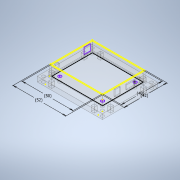
# Autodesk Inventor part: TNC Case
Saved by Autodesk Inventor 2020.1 (Build 241239000, 239)
## iProperties
Created: 2019-09-18
Part Number: TNC Case
Material: PET Plastic
Document SubType Name: Modeling
Designer: Logan
Density: 1.541 g/cm^3
Appearance: Polycarbonate - Clear
Author: Logan
Autodesk Inventor part; units mm, degrees
ref_plane "YZ Plane" through (0, 0, 0) normal (1, 0, 0) x (0, 1, 0)
ref_plane "XZ Plane" through (0, 0, 0) normal (0, 1, 0) x (-1, 0, 0)
ref_plane "XY Plane" through (0, 0, 0) normal (0, 0, 1) x (1, 0, 0)
sketch "Sketch1" plane through (0, 0, 0) normal (0, 1, 0) x (-1, 0, 0)
  line L0 (0, 0) -> (60, 0)
  line L1 (60, 0) -> (60, -50)
  line L2 (60, -50) -> (0, -50)
  line L3 (0, -50) -> (0, 0)
  line L4 (60, 0) -> (0, 0)
  line L5 (0, 0) -> (0, -5)
  line L6 (0, -5) -> (60, -5)
  line L7 (60, -5) -> (60, 0)
  line L8 (60, 0) -> (55, 0)
  line L9 (55, 0) -> (55, -50)
  line L10 (55, -50) -> (60, -50)
  line L11 (60, -50) -> (60, 0)
  line L12 (60, -50) -> (0, -50)
  line L13 (0, -50) -> (0, -45)
  line L14 (0, -45) -> (60, -45)
  line L15 (60, -45) -> (60, -50)
  line L16 (0, -50) -> (5, -50)
  line L17 (5, -50) -> (5, 0)
  line L18 (5, 0) -> (0, 0)
  line L19 (0, 0) -> (0, -50)
  line L20 (5, -5) -> (55, -5)
  line L21 (55, -5) -> (55, -45)
  line L22 (55, -45) -> (5, -45)
  line L23 (5, -45) -> (5, -5)
  dimension "d0" = 60
  dimension "d1" = 50
  dimension "d2" = 5
  dimension "d3" = 5
  dimension "d4" = 5
  dimension "d5" = 5
  dimension "d6" = 40
  dimension "d7" = 50
  constraints: 48 end point, 12 parallel, 8 point on line, 6 horizontal, 6 perpendicular
  measures "d0" distance of L1.end L2.end
  measures "d1" distance of L0.end L1.end
  measures "d2" distance of L5.end L4.end
  measures "d3" distance of L10.end L9.end
  measures "d4" distance of L12.end L13.end
  measures "d5" distance of L18.end L17.end
  measures "d6" distance between parallel lines of L22 L20
  measures "d7" distance between parallel lines of L23 L21
extrude "Extrusion1" add sketch "Sketch1" along normal blind 5
sketch "Sketch2" plane through (0, 5, 0) normal (0, 1, 0) x (1, 0, 0)
  line L0 (-60, 50) -> (-60, 0) projected
  line L1 (0, 50) -> (-60, 50) projected
  line L2 (-60, 0) -> (0, 0)
  line L3 (0, 0) -> (0, 50)
  line L4 (0, 50) -> (-60, 50)
  line L5 (-60, 50) -> (-60, 0)
  line L6 (0, 0) -> (0, 50) projected
  line L7 (-60, 0) -> (0, 0)
  line L8 (0, 0) -> (0, 5)
  line L9 (0, 5) -> (-60, 5)
  line L10 (-60, 5) -> (-60, 0)
  line L11 (0, 50) -> (-60, 50)
  line L12 (-60, 50) -> (-60, 45)
  line L13 (-60, 45) -> (0, 45)
  line L14 (0, 45) -> (0, 50)
  line L15 (-60, 0) -> (0, 0) projected
  line L16 (-60, 50) -> (-55, 50)
  line L17 (-55, 50) -> (-55, 0)
  line L18 (-55, 0) -> (-60, 0)
  line L19 (-60, 0) -> (-60, 50)
  line L20 (0, 0) -> (-5, 0)
  line L21 (-5, 0) -> (-5, 50)
  line L22 (-5, 50) -> (0, 50)
  line L23 (0, 50) -> (0, 0)
  line L24 (-55, 5) -> (-56.5, 5)
  line L25 (-56.5, 5) -> (-56.5, 3.5)
  line L26 (-56.5, 3.5) -> (-55, 3.5)
  line L27 (-55, 3.5) -> (-55, 5)
  line L28 (-60, 0) -> (-62, 0)
  line L29 (-62, 0) -> (-62, 50)
  line L30 (-62, 50) -> (-60, 50)
  line L31 (-60, 50) -> (-60, 0)
  line L32 (-62, 0) -> (0, 0)
  line L33 (0, 0) -> (0, -2)
  line L34 (0, -2) -> (-62, -2)
  line L35 (-62, -2) -> (-62, 0)
  line L36 (-62, 50) -> (2, 50)
  line L37 (2, 50) -> (2, 52)
  line L38 (2, 52) -> (-62, 52)
  line L39 (-62, 52) -> (-62, 50)
  line L40 (2, 50) -> (0, 50)
  line L41 (0, 50) -> (0, -2)
  line L42 (0, -2) -> (2, -2)
  line L43 (2, -2) -> (2, 50)
  dimension "d10" = 5
  dimension "d11" = 5
  dimension "d12" = 5
  dimension "d13" = 5
  dimension "d14" = 1.5
  dimension "d15" = 1.5
  dimension "d16" = 2
  dimension "d17" = 2
  dimension "d18" = 64
  dimension "d19" = 2
  constraints: 80 end point, 20 parallel, 10 horizontal, 10 perpendicular, 8 point on line
  measures "d10" distance of L8.end L7.end
  measures "d11" distance of L12.end L11.end
  measures "d12" distance of L17.end L18.end
  measures "d13" distance of L21.end L22.end
  measures "d14" distance of L26.end L25.end
  measures "d15" distance of L25.end L24.end
  measures "d16" distance of L29.end L30.end
  measures "d17" distance of L32.end L33.end
  measures "d18" distance of L38.end L37.end
  measures "d19" distance of L37.end L36.end
extrude "Extrusion2" add sketch "Sketch2" against normal blind 5 contours L30 L39 L38 L37 L36 L1 | L0 L28 L29 L30 | L28 L2 L33 L34 L35 | L36 L43 L42 L33 L3
sketch "Sketch3" plane through (0, 5, 0) normal (0, 1, 0) x (1, 0, 0)
  line L0 (2, -2) -> (-62, -2) projected
  line L1 (2, 52) -> (2, -2) projected
  line L2 (-62, -2) -> (2, -2)
  line L3 (2, -2) -> (2, 52)
  line L4 (2, 52) -> (-62, 52)
  line L5 (-62, 52) -> (-62, -2)
  line L6 (-62, -2) -> (2, -2)
  line L7 (2, -2) -> (2, 4)
  line L8 (2, 4) -> (-62, 4)
  line L9 (-62, 4) -> (-62, -2)
  line L10 (2, 52) -> (-62, 52)
  line L11 (-62, 52) -> (-62, 46)
  line L12 (-62, 46) -> (2, 46)
  line L13 (2, 46) -> (2, 52)
  line L14 (-62, -2) -> (-62, 52) projected
  line L15 (-62, 52) -> (-56, 52)
  line L16 (-56, 52) -> (-56, -2)
  line L17 (-56, -2) -> (-62, -2)
  line L18 (-62, -2) -> (-62, 52)
  line L19 (-62, 52) -> (2, 52) projected
  line L20 (2, -2) -> (-4, -2)
  line L21 (-4, -2) -> (-4, 52)
  line L22 (-4, 52) -> (2, 52)
  line L23 (2, 52) -> (2, -2)
  line L24 (-4, 46) -> (-54, 46)
  line L25 (-54, 46) -> (-54, 6)
  line L26 (-54, 6) -> (-4, 6)
  line L27 (-4, 6) -> (-4, 46)
  line L28 (-56, 4) -> (-6, 4)
  line L29 (-6, 4) -> (-6, 44)
  line L30 (-6, 44) -> (-56, 44)
  line L31 (-56, 44) -> (-56, 4)
  line L32 (-56, 4) -> (-5, 4)
  line L33 (-5, 4) -> (-5, 45)
  line L34 (-5, 45) -> (-56, 45)
  line L35 (-56, 45) -> (-56, 4)
  line L36 (-4, 46) -> (-55, 46)
  line L37 (-55, 46) -> (-55, 5)
  line L38 (-55, 5) -> (-4, 5)
  line L39 (-4, 5) -> (-4, 46)
  line L40 (-4, 5) -> (-56, 5)
  line L41 (-56, 5) -> (-56, 4)
  line L42 (-56, 4) -> (-4, 4)
  line L43 (-4, 4) -> (-4, 5)
  line L44 (-56, 4) -> (-55, 4)
  line L45 (-55, 4) -> (-55, 46)
  line L46 (-55, 46) -> (-56, 46)
  line L47 (-56, 46) -> (-56, 4)
  line L48 (-56, 45) -> (-4, 45)
  line L49 (-4, 45) -> (-4, 46)
  line L50 (-4, 46) -> (-56, 46)
  line L51 (-56, 46) -> (-56, 45)
  line L52 (-4, 46) -> (-5, 46)
  line L53 (-5, 46) -> (-5, 4)
  line L54 (-5, 4) -> (-4, 4)
  line L55 (-4, 4) -> (-4, 46)
  point P0 (0, 0)
  point P1 (-4, 4)
  point P2 (-55, 45)
  point P3 (-5, 5)
  point P4 (-55, 5)
  dimension "d22" = 6
  dimension "d23" = 6
  dimension "d24" = 6
  dimension "d25" = 6
  dimension "d26" = 50
  dimension "d27" = 40
  dimension "d28" = 50
  dimension "d29" = 40
  dimension "d30" = 51
  dimension "d31" = 41
  dimension "d32" = 51
  dimension "d33" = 41
  dimension "d34" = 40
  dimension "d35" = 50
  constraints: 104 end point, 26 parallel, 13 horizontal, 13 perpendicular, 8 point on line
  measures "d22" distance of L7.end L6.end
  measures "d23" distance of L11.end L10.end
  measures "d24" distance of L16.end L17.end
  measures "d25" distance of L21.end L22.end
  measures "d26" distance of L26.end L25.end
  measures "d27" distance of L25.end L24.end
  measures "d28" distance of L30.end L29.end
  measures "d29" distance of L29.end L28.end
  measures "d30" distance of L34.end L33.end
  measures "d31" distance of L33.end L32.end
  measures "d32" distance of L38.end L37.end
  measures "d33" distance of L37.end L36.end
  measures "d34" distance between parallel lines of L34 L38
  measures "d35" distance between parallel lines of L33 L37
extrude "Extrusion3" add sketch "Sketch3" along normal blind 10 contours L8 L33 L38 L21 | L16 L40 L45 L8 | L8 L29 L38 L33 | L38 L33 L26 L21 | L21 L48 L53 L12 | L45 L38 L29 L8 | L16 L30 L37 L40 | L26 L33 L48 L21 | L53 L34 L25 L12 | L16 L34 L37 L30 | L25 L34 L37 L12 | L12 L37 L34 L16
sketch "Sketch5" plane through (0, 5, 0) normal (0, 1, 0) x (1, 0, 0)
  line L0 (-55, 5) -> (-55, 45) projected
  line L1 (-55, 45) -> (-5, 45) projected
  line L2 (-55, 5) -> (-5, 5)
  line L3 (-5, 5) -> (-5, 45)
  line L4 (-5, 45) -> (-55, 45)
  line L5 (-55, 45) -> (-55, 5)
  line L6 (-55, 5) -> (-51, 5)
  line L7 (-55, 9) -> (-55, 5)
  circle A0 centre (-51, 9) radius 1.5
  line L8 (-5, 45) -> (-5, 5) projected
  line L9 (-5, 5) -> (-9, 5)
  line L10 (-5, 9) -> (-5, 5)
  line L11 (-5, 45) -> (-9, 45)
  line L12 (-5, 41) -> (-5, 45)
  line L13 (-55, 45) -> (-51, 45)
  line L14 (-55, 41) -> (-55, 45)
  circle A1 centre (-9, 41) radius 1.5
  circle A2 centre (-9, 9) radius 1.5
  point P0 (0, 0)
  constraints: 24 end point, 5 horizontal, 3 centre point, 2 parallel, 1 perpendicular
extrude "Extrusion4" cut sketch "Sketch5" against normal blind 10 contours A0 | A1 | A2
sketch "Sketch6" plane through (-4, 5, -4) normal (1, 0, 0) x (0, 0, -1)
  line L0 (0, 10) -> (1, 10)
  line L1 (1, 10) -> (1, 0)
  line L2 (1, 0) -> (0, 0)
  line L3 (0, 0) -> (0, 10)
  line L4 (41, 10) -> (42, 10)
  line L5 (42, 10) -> (42, 0)
  line L6 (42, 0) -> (41, 0)
  line L7 (41, 0) -> (41, 10)
  line L8 (1, 0) -> (6, 0)
  line L9 (6, 0) -> (6, 2)
  line L10 (1, 2) -> (1, 0)
  line L11 (6, 2) -> (24, 2)
  line L12 (24, 2) -> (24, 0)
  line L13 (24, 0) -> (6, 0)
  line L14 (6, 0) -> (6, 2)
  line L15 (1, 0) -> (41, 0) projected
  line L16 (6, 2) -> (11.05, 2)
  line L17 (11.05, 0) -> (6, 0)
  line L18 (6, 0) -> (6, 2)
  line L19 (24, 0) -> (18.95, 0)
  line L20 (18.95, 2) -> (24, 2)
  line L21 (24, 2) -> (24, 0)
  line L22 (6, 2) -> (15, 2)
  line L23 (15, 2) -> (15, 0)
  line L24 (15, 0) -> (6, 0)
  line L25 (6, 0) -> (6, 2)
  line L26 (24, 0) -> (15, 0)
  line L27 (15, 0) -> (15, 2)
  line L28 (15, 2) -> (24, 2)
  line L29 (24, 2) -> (24, 0)
  line L30 (15, 2) -> (12.525, 2)
  line L31 (12.525, 2) -> (12.525, 0)
  line L32 (12.525, 0) -> (15, 0)
  line L33 (15, 0) -> (15, 2)
  line L34 (15, 2) -> (17.475, 2)
  line L35 (17.475, 2) -> (17.475, 0)
  line L36 (17.475, 0) -> (15, 0)
  line L37 (15, 0) -> (15, 2)
  line L38 (24, 0) -> (24.05, 0)
  line L39 (24.05, 0) -> (24.05, 2)
  line L40 (24, 2) -> (24, 0)
  line L41 (24.05, 2) -> (31.55, 2)
  line L42 (31.55, 2) -> (31.55, 0)
  line L43 (31.55, 0) -> (24.05, 0)
  line L44 (24.05, 0) -> (24.05, 2)
  line L45 (32.05, 2) -> (32.05, 0)
  line L46 (32.05, 0) -> (31.55, 0)
  line L47 (31.55, 0) -> (31.55, 2)
  line L48 (32.05, 0) -> (37.05, 0)
  line L49 (37.05, 0) -> (37.05, 2)
  line L50 (37.05, 2) -> (32.05, 2)
  line L51 (32.05, 2) -> (32.05, 0)
  line L52 (1, 0) -> (1, 10) projected
  line L53 (41, 0) -> (1, 0)
  line L54 (1, 0) -> (1, 1.6)
  line L55 (1, 1.6) -> (41, 1.6)
  line L56 (41, 1.6) -> (41, 0)
  line L57 (37.05, 2) -> (32.05, 2)
  line L58 (32.05, 2) -> (32.05, 1.6)
  line L59 (32.05, 1.6) -> (37.05, 1.6)
  line L60 (37.05, 1.6) -> (37.05, 2)
  line L61 (37.05, 2) -> (32.05, 2)
  line L62 (32.05, 2) -> (32.05, 1.6)
  line L63 (32.05, 1.6) -> (37.05, 1.6)
  line L64 (37.05, 1.6) -> (37.05, 2)
  line L65 (37.05, 1.6) -> (32.05, 1.6)
  line L66 (32.05, 1.6) -> (32.05, 6.6)
  line L67 (32.05, 6.6) -> (37.05, 6.6)
  line L68 (37.05, 6.6) -> (37.05, 1.6)
  line L69 (17.475, 2) -> (12.525, 2)
  line L70 (12.525, 2) -> (12.525, 1.6)
  line L71 (12.525, 1.6) -> (17.475, 1.6)
  line L72 (17.475, 1.6) -> (17.475, 2)
  line L73 (15, 1.6) -> (17.57, 1.6)
  line L74 (17.57, 1.6) -> (17.57, 2)
  line L75 (17.57, 2) -> (15, 2)
  line L76 (15, 2) -> (15, 1.6)
  line L77 (15, 1.6) -> (12.43, 1.6)
  line L78 (12.43, 1.6) -> (12.43, 2)
  line L79 (12.43, 2) -> (15, 2)
  line L80 (15, 2) -> (15, 1.6)
  line L81 (17.57, 1.6) -> (12.43, 1.6)
  line L82 (12.43, 1.6) -> (12.43, 8.15)
  line L83 (12.43, 8.15) -> (17.57, 8.15)
  line L84 (17.57, 8.15) -> (17.57, 1.6)
  line L85 (31.55, 1.6) -> (24.05, 1.6)
  line L86 (24.05, 1.6) -> (24.05, 6.6)
  line L87 (24.05, 6.6) -> (31.55, 6.6)
  line L88 (31.55, 6.6) -> (31.55, 1.6)
  point P0 (-4, -5)
  point P1 (32.05, 2)
  point P2 (37.05, 2)
  point P3 (24.05, 2)
  point P4 (31.55, 2)
  point P5 (12.43, 2)
  point P6 (17.57, 2)
  dimension "d48" = 5.05
  dimension "d53" = 7.5
  dimension "d54" = 0.5
  dimension "d55" = 5
  dimension "d58" = 1.6
  dimension "d59" = 5
  dimension "d60" = 5
  dimension "d61" = 2.57
  dimension "d62" = 2.57
  dimension "d63" = 6.55
  dimension "d64" = 7.5
  constraints: 174 end point, 41 parallel, 22 horizontal, 20 perpendicular, 12 point on line, 1 midpoint, 5 other
  measures "d48" distance of L20.start L20.end
  measures "d53" distance of L42.end L43.end
  measures "d54" distance of L45.end L46.end
  measures "d55" distance of L50.end L49.end
  measures "d58" distance of L53.end L54.end
  measures "d59" distance of L66.end L67.end
  measures "d60" distance of L65.end L66.end
  measures "d61" distance of L75.end L74.end
  measures "d62" distance of L78.end L79.end
  measures "d63" distance of L81.end L82.end
  measures "d64" distance of L86.end L87.end
sketch "Sketch7" plane through (0, 5, 0) normal (0, 1, 0) x (1, 0, 0)
  point P0 (0, 0)
sketch "Sketch8" plane through (0, 5, 0) normal (0, 1, 0) x (1, 0, 0)
  line L0 (-55, 5) -> (-5, 5) projected
  line L1 (-5, 45) -> (-55, 45) projected
  line L2 (-5, 5) -> (-55, 5)
  line L3 (-55, 5) -> (-55, 45)
  line L4 (-55, 45) -> (-5, 45)
  line L5 (-5, 45) -> (-5, 5)
  circle A0 centre (-51, 9) radius 1.5
  circle A1 centre (-9, 9) radius 1.5
  circle A2 centre (-9, 41) radius 1.5 projected
  circle A3 centre (-9, 41) radius 1.5
  point P0 (0, 0)
  constraints: 8 end point, 3 centre point, 2 parallel, 1 coincident, 1 horizontal, 1 perpendicular
sketch "Sketch9" plane through (-4, 5, -4) normal (1, 0, 0) x (0, 0, -1)
  point P0 (-4, -5)
extrude "Extrusion6" cut sketch "Sketch6" against normal blind 10 contours L82 L83 L84 L11 | L86 L87 L88 L41 | L66 L67 L68 L50
sketch "Sketch10" plane through (-56, 5, -46) normal (-1, 0, 0) x (0, 0, 1)
  point P0 (46, -5)
  point P1 (0, 10)
  point P2 (42, 0)
  point P3 (41, 10)
sketch "Sketch11" plane through (-56, 5, -46) normal (-1, 0, 0) x (0, 0, 1)
  line L0 (2, 1.6) -> (8.3, 1.6)
  line L1 (8.3, 1.6) -> (8.3, 7.9)
  line L2 (8.3, 7.9) -> (2, 7.9)
  line L3 (2, 7.9) -> (2, 1.6)
  point P0 (46, -5)
  constraints: 8 end point, 2 parallel, 1 horizontal, 1 perpendicular
extrude "Extrusion7" cut sketch "Sketch11" against normal blind 10
extrude "Extrusion8" cut sketch "Sketch11" against normal blind 10
sketch "Sketch12" plane through (-56, 5, -46) normal (-1, 0, 0) x (0, 0, 1)
  line L0 (42, 0) -> (42, 10) projected
  line L1 (42, 1.5824) -> (0, 1.5824)
  line L2 (0, 1.5824) -> (0, 10)
  line L3 (0, 10) -> (42, 10)
  line L4 (42, 10) -> (42, 1.5824)
  line L5 (41, 10) -> (1, 10) projected
  line L6 (42, 1.5824) -> (35.5, 1.5824)
  line L7 (35.5, 1.5824) -> (35.5, 10)
  line L8 (35.5, 10) -> (42, 10)
  line L9 (42, 10) -> (42, 1.5824)
  circle A0 centre (35.5, 5.7912) radius 2.5
  point P0 (46, -5)
  dimension "d74" = 6.5
  dimension "d75" = 5
  constraints: 16 end point, 4 parallel, 2 horizontal, 2 perpendicular, 2 point on line, 1 centre point, 1 midpoint
  measures "d74" distance of L7.end L8.end
  measures "d75" diameter of A0
extrude "Extrusion9" cut sketch "Sketch12" against normal blind 10 contours A0 L7 | L7 A0
sketch "Sketch13" plane through (0, 5, 0) normal (0, 1, 0) x (1, 0, 0)
  line L0 (2, 52) -> (2, -2) projected
  line L1 (2, -2) -> (-4, -2)
  line L2 (-4, -2) -> (-4, 4)
  line L3 (-4, 4) -> (2, 4)
  line L4 (2, 4) -> (2, -2)
  line L5 (2, -2) -> (-1, -2)
  line L6 (-1, -2) -> (-1, 1)
  line L7 (-1, 1) -> (2, 1)
  line L8 (2, 1) -> (2, -2)
  circle A0 centre (-1, 1) radius 1.5
  line L9 (2, 52) -> (-4, 52)
  line L10 (-4, 52) -> (-4, 46)
  line L11 (-4, 46) -> (2, 46)
  line L12 (2, 46) -> (2, 52)
  line L13 (2.2559, 52) -> (-0.7441, 52)
  line L14 (-0.7441, 52) -> (-0.7441, 49)
  line L15 (-0.7441, 49) -> (2.2559, 49)
  line L16 (2.2559, 49) -> (2.2559, 52)
  circle A1 centre (-0.7441, 49) radius 1.5
  line L17 (-56, 4) -> (-56, 46) projected
  line L18 (-62, 52) -> (-56, 52)
  line L19 (-56, 52) -> (-56, 46)
  line L20 (-56, 46) -> (-62, 46)
  line L21 (-62, 46) -> (-62, 52)
  line L22 (2, 52) -> (-62, 52) projected
  line L23 (-62, 52) -> (-59, 52)
  line L24 (-59, 52) -> (-59, 49)
  line L25 (-59, 49) -> (-62, 49)
  line L26 (-62, 49) -> (-62, 52)
  circle A2 centre (-59, 49) radius 1.5
  circle A3 centre (-59, 1) radius 1.5
  circle A4 centre (-51, 9) radius 1.5 projected
  line L27 (-51, 10.5) -> (-60.5, 10.5)
  line L28 (-60.5, 10.5) -> (-60.5, 7.5)
  line L29 (-60.5, 7.5) -> (-51, 7.5)
  line L30 (-51, 7.5) -> (-51, 10.5)
  line L31 (-52.4117, 9) -> (-49.4117, 9)
  line L32 (-49.4117, 9) -> (-49.4117, -0.5)
  line L33 (-49.4117, -0.5) -> (-52.4117, -0.5)
  line L34 (-52.4117, -0.5) -> (-52.4117, 9)
  line L35 (-49.4117, -0.5) -> (-52.4117, -0.5)
  line L36 (-52.4117, -0.5) -> (-52.4117, 2.5)
  line L37 (-52.4117, 2.5) -> (-49.4117, 2.5)
  line L38 (-49.4117, 2.5) -> (-49.4117, -0.5)
  line L39 (-60.5, 7.5) -> (-57.5, 7.5)
  line L40 (-57.5, 7.5) -> (-57.5, 10.5)
  line L41 (-57.5, 10.5) -> (-60.5, 10.5)
  line L42 (-60.5, 10.5) -> (-60.5, 7.5)
  circle A5 centre (-9, 9) radius 1.5 projected
  line L43 (-9, 7.5) -> (0.5, 7.5)
  line L44 (0.5, 7.5) -> (0.5, 10.5)
  line L45 (0.5, 10.5) -> (-9, 10.5)
  line L46 (-9, 10.5) -> (-9, 7.5)
  line L47 (-7.5, 9) -> (-10.5, 9)
  line L48 (-10.5, 9) -> (-10.5, -0.5)
  line L49 (-10.5, -0.5) -> (-7.5, -0.5)
  line L50 (-7.5, -0.5) -> (-7.5, 9)
  circle A6 centre (-9, 41) radius 1.5 projected
  line L51 (-9, 39.5) -> (0, 39.5)
  line L52 (0, 39.5) -> (0, 42.5)
  line L53 (0, 42.5) -> (-9, 42.5)
  line L54 (-9, 42.5) -> (-9, 39.5)
  line L55 (1, 42.5) -> (-9, 42.5)
  line L56 (-9, 42.5) -> (-9, 39.5)
  line L57 (-9, 39.5) -> (1, 39.5)
  line L58 (1, 39.5) -> (1, 42.5)
  line L59 (1, 10.5) -> (-9, 10.5)
  line L60 (-9, 10.5) -> (-9, 7.5)
  line L61 (-9, 7.5) -> (1, 7.5)
  line L62 (1, 7.5) -> (1, 10.5)
  line L63 (-7.5, 41) -> (-10.5, 41)
  line L64 (-10.5, 41) -> (-10.5, 50.5)
  line L65 (-10.5, 50.5) -> (-7.5, 50.5)
  line L66 (-7.5, 50.5) -> (-7.5, 41)
  circle A7 centre (-50.9117, 41) radius 1.5
  line L67 (-50.9117, 39.5) -> (-60.5, 39.5)
  line L68 (-60.5, 39.5) -> (-60.5, 42.5)
  line L69 (-60.5, 42.5) -> (-50.9117, 42.5)
  line L70 (-50.9117, 42.5) -> (-50.9117, 39.5)
  line L71 (-52.4117, 41) -> (-49.4117, 41)
  line L72 (-49.4117, 41) -> (-49.4117, 50.5)
  line L73 (-49.4117, 50.5) -> (-52.4117, 50.5)
  line L74 (-52.4117, 50.5) -> (-52.4117, 41)
  line L75 (-60.5, 39.5) -> (-57.5, 39.5)
  line L76 (-57.5, 39.5) -> (-57.5, 42.5)
  line L77 (-57.5, 42.5) -> (-60.5, 42.5)
  line L78 (-60.5, 42.5) -> (-60.5, 39.5)
  line L79 (-49.4117, 50.5) -> (-52.4117, 50.5)
  line L80 (-52.4117, 50.5) -> (-52.4117, 47.5)
  line L81 (-52.4117, 47.5) -> (-49.4117, 47.5)
  line L82 (-49.4117, 47.5) -> (-49.4117, 50.5)
  line L83 (-7.5, 50.5) -> (-10.5, 50.5)
  line L84 (-10.5, 50.5) -> (-10.5, 47.5)
  line L85 (-10.5, 47.5) -> (-7.5, 47.5)
  line L86 (-7.5, 47.5) -> (-7.5, 50.5)
  line L87 (-2.2441, 42.5) -> (0.7559, 42.5)
  line L88 (0.7559, 42.5) -> (0.7559, 39.5)
  line L89 (0.7559, 39.5) -> (-2.2441, 39.5)
  line L90 (-2.2441, 39.5) -> (-2.2441, 42.5)
  line L91 (-2.5, 7.5) -> (0.5, 7.5)
  line L92 (0.5, 7.5) -> (0.5, 10.5)
  line L93 (0.5, 10.5) -> (-2.5, 10.5)
  line L94 (-2.5, 10.5) -> (-2.5, 7.5)
  line L95 (-7.5, -0.5) -> (-10.5, -0.5)
  line L96 (-10.5, -0.5) -> (-10.5, 2.5)
  line L97 (-10.5, 2.5) -> (-7.5, 2.5)
  line L98 (-7.5, 2.5) -> (-7.5, -0.5)
  point P0 (0, 0)
  dimension "d78" = 3
  dimension "d79" = 3
  dimension "d80" = 3
  dimension "d81" = 3
  dimension "d82" = 3
  dimension "d83" = 3
  dimension "d84" = 3
  dimension "d85" = 3
  dimension "d86" = 3
  constraints: 192 end point, 48 parallel, 24 horizontal, 24 perpendicular, 14 point on line, 6 point on circle, 5 centre point, 3 coincident, 1 vertical alignment, 1 other
  measures "d78" diameter of A0
  measures "d79" distance of L15.end L14.end
  measures "d80" distance of L14.end L13.end
  measures "d81" diameter of A1
  measures "d82" distance of L24.end L25.end
  measures "d83" diameter of A2
  measures "d84" diameter of A3
  measures "d85" distance of L32.end L33.end
  measures "d86" distance of L88.end L89.end
extrude "Extrusion10" cut sketch "Sketch13" against normal blind 10 contours A1 L14 L15 | L15 L14 A1 | A0 L6 L7 | L7 L6 A0 | A2 L25 L24 | L24 L25 A2 | L76 L67 L68 L69 | L74 L73 L72 L81 | L40 L29 L28 L27 | L37 L32 L33 L34 | A3 | L45 L44 L43 L94 | L50 L49 L48 L97 | L90 L53 L52 L51 | L85 L64 L65 L66 | L52 L55 L88 L57
sketch "Sketch14" plane through (0, 15, 0) normal (0, 1, 0) x (1, 0, 0)
  line L0 (-55, 45) -> (-5, 45) projected
  line L1 (-5, 5) -> (-55, 5) projected
  line L2 (-5, 45) -> (-5, 5) projected
  line L3 (-55, 5) -> (-55, 45) projected
  line L4 (-4, 4) -> (-4, 46) projected
  line L5 (-56, 46) -> (-56, 4) projected
  line L6 (-4, 46) -> (-56, 46) projected
  line L7 (-56, 4) -> (-4, 4) projected
  point P0 (0, 0)
  dimension "d89" = 40
  dimension "d90" = 50
  dimension "d91" = 52
  dimension "d92" = 42
  measures "d89" distance between parallel lines of L0 L1
  measures "d90" distance between parallel lines of L2 L3
  measures "d91" distance between parallel lines of L4 L5
  measures "d92" distance between parallel lines of L6 L7
body "Solid1"
